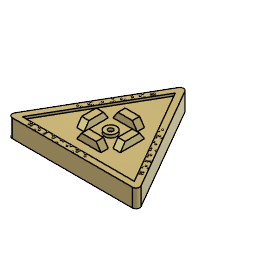
Piece Gold Minefinalweb (Autodesk Fusion 360 design; units mm, degrees)
Autodesk Fusion 360 part; units mm, degrees
note: some values were not read from the file. Set by a fixed rule: which sketch regions a step uses.
sketch "Sketch1" plane through (0, 0, 0) normal (0, 1, 0) x (1, 0, 0) in component "Goldmine"
  line L0 (0, 0) -> (69.85, 120.9837)
  line L1 (0, 0) -> (139.7, 0)
  line L2 (69.85, 120.9837) -> (139.7, 0)
  dimension "d1" = 139.7
  dimension "d2" = 139.7
  dimension "d4" = 139.7
  constraint coincident L0.start L1.start
  constraint horizontal L1
  measures "d1" distance of L0.start L0.end
  measures "d2" distance of L0.start L1.end
  measures "d4" distance of L0.end L1.end
extrude "Extrude1" add sketch "Sketch1" along normal blind 19.05 in component "Goldmine"
sketch "Sketch5" plane through (0, 19.05, 0) normal (0, 1, 0) x (-1, 0, 0) in component "Goldmine"
  line L0 (0, 0) -> (-139.7, 0)
  line L1 (-139.7, 0) -> (-69.85, -120.9837)
  line L2 (-69.85, -120.9837) -> (0, 0)
  line L3 (-10.9985, -6.35) -> (-69.85, -108.2837)
  line L4 (-69.85, -108.2837) -> (-128.7015, -6.35)
  line L5 (-128.7015, -6.35) -> (-10.9985, -6.35)
  dimension "d65" = 6.35
  dimension "d66" = 6.35
  dimension "d67" = 6.35
  constraint parallel L2 L3
  constraint parallel L1 L4
  constraint parallel L0 L5
  measures "d65" distance of L0 L3.start
  measures "d66" distance of L2 L3
  measures "d67" distance of L1 L4
extrude "Extrude6" cut sketch "Sketch5" against normal blind 2.54 contours L3 L4 L5 in component "Goldmine"
ref_plane "WorkPlane1" through (50.8, 0, 0) normal (1, 0, 0) x (0, 1, 0) in component "Goldmine"
sketch "Sketch10" plane through (0, 16.51, 0) normal (0, 1, 0) x (-1, 0, 0) in component "Goldmine"
  line L0 (-128.7015, -6.35) -> (-69.85, -108.2837)
  line L1 (-69.85, -108.2837) -> (-10.9985, -6.35)
  line L2 (-10.9985, -6.35) -> (-128.7015, -6.35)
  circle A0 centre (-69.85, -40.3279) radius 6.35
  circle A1 centre (-69.85, -40.3279) radius 2.54
  line L3 (-69.85, -40.3279) -> (-69.85, -108.2837) construction
  line L4 (-69.85, -40.3279) -> (-10.9985, -6.35) construction
  line L5 (-69.85, -40.3279) -> (-128.7015, -6.35) construction
  point P0 (-69.85, -108.2837)
  point P1 (-10.9985, -6.35)
  point P2 (-128.7015, -6.35)
  dimension "d125" = 12.7
  dimension "d126" = 5.08
  constraint concentric A0 A1
  constraint coincident A0.centre A1.centre
  constraint coincident P0 L0.end
  constraint coincident P1 L1.end
  constraint coincident P2 L0.start
  constraint equal L3 L4
  constraint equal L4 L5
  measures "d125" diameter of A0
  measures "d126" diameter of A1
extrude "Extrude14" add sketch "Sketch10" along normal blind 3.048 contours A0 in component "Goldmine"
sketch "Sketch11" plane through (0, 16.51, 0) normal (0, 1, 0) x (-1, 0, 0) in component "Goldmine"
  line L0 (-128.7015, -6.35) -> (-69.85, -108.2837)
  line L1 (-10.9985, -6.35) -> (-128.7015, -6.35)
  circle A0 centre (-69.85, -40.3279) radius 6.35
  circle A1 centre (-69.85, -40.3279) radius 2.54
  line L2 (-46.99, -53.0279) -> (-54.61, -53.0279)
  line L3 (-54.61, -53.0279) -> (-54.61, -27.6279)
  line L4 (-54.61, -27.6279) -> (-46.99, -27.6279)
  line L5 (-46.99, -27.6279) -> (-46.99, -53.0279)
  line L6 (-85.09, -53.0279) -> (-92.71, -53.0279)
  line L7 (-92.71, -53.0279) -> (-92.71, -27.6279)
  line L8 (-92.71, -27.6279) -> (-85.09, -27.6279)
  line L9 (-85.09, -27.6279) -> (-85.09, -53.0279)
  line L10 (-57.15, -63.1879) -> (-82.55, -63.1879)
  line L11 (-82.55, -63.1879) -> (-82.55, -55.5679)
  line L12 (-82.55, -25.0879) -> (-82.55, -17.4679)
  line L13 (-82.55, -17.4679) -> (-57.15, -17.4679)
  line L14 (-57.15, -63.1879) -> (-57.15, -55.5679)
  line L15 (-57.15, -55.5679) -> (-82.55, -55.5679)
  line L16 (-82.55, -25.0879) -> (-57.15, -25.0879)
  line L17 (-57.15, -25.0879) -> (-57.15, -17.4679)
  dimension "d129" = 25.4
  dimension "d130" = 7.62
  dimension "d131" = 15.24
  dimension "d132" = 12.7
  dimension "d133" = 7.62
  dimension "d134" = 25.4
  dimension "d135" = 30.48
  dimension "d152" = 2.54
  dimension "d153" = 7.62
  dimension "d154" = 25.4
  dimension "d155" = 7.62
  dimension "d156" = 15.24
  dimension "d157" = 2.54
  dimension "d158" = 7.62
  dimension "d159" = 25.4
  dimension "d160" = 15.24
  dimension "d161" = 2.54
  constraint horizontal L2
  constraint vertical L3
  constraint horizontal L4
  constraint vertical L5
  constraint horizontal L6
  constraint vertical L7
  constraint horizontal L8
  constraint vertical L9
  constraint horizontal L2.end L6.start
  constraint horizontal L10
  constraint vertical L11
  constraint vertical L12
  constraint horizontal L13
  constraint perpendicular L10 L14
  constraint perpendicular L3 L16
  constraint perpendicular L13 L17
  measures "d129" distance of L2.start L4.end
  measures "d130" distance of L3.end L4.end
  measures "d131" distance of A0.centre L3
  measures "d132" distance of A0.centre L2
  measures "d133" distance of L6.start L6.end
  measures "d134" distance of L6.start L8.end
  measures "d135" distance of L3 L9
  measures "d152" horizontal distance of L6.start L11.end
  measures "d153" distance of L10.end L11.end
  measures "d154" distance of L10.start L10.end
  measures "d155" distance of L10.start L14.end
  measures "d156" distance of A0.centre L15
  measures "d157" horizontal distance of L8.end L12.start
  measures "d158" distance of L12.start L12.end
  measures "d159" distance of L12.start L16.end
  measures "d160" vertical distance of A0.centre L16.end
  measures "d161" vertical distance of L8.end L12.start
extrude "Extrude15" add sketch "Sketch11" along normal blind 7.62 contours L2 L3 L4 L5 | L6 L7 L8 L9 | L10 L11 L14 L15 | L12 L13 L16 L17 in component "Goldmine"
sketch "Sketch12" plane through (92.71, 0, 0) normal (1, 0, 0) x (0, 0, -1) in component "Goldmine"
  line L0 (27.6279, 16.51) -> (53.0279, 16.51)
  line L1 (53.0279, 16.51) -> (53.0279, 24.13)
  line L2 (53.0279, 24.13) -> (27.6279, 24.13)
  line L3 (27.6279, 24.13) -> (27.6279, 16.51)
  line L4 (27.6279, 16.51) -> (32.7079, 24.13)
  line L5 (27.6279, 24.13) -> (27.6279, 16.51)
  line L6 (32.7079, 24.13) -> (27.6279, 24.13)
  line L7 (53.0279, 16.51) -> (47.9479, 24.13)
  line L8 (53.0279, 24.13) -> (47.9479, 24.13)
  line L9 (53.0279, 24.13) -> (53.0279, 16.51)
  dimension "d144" = 5.08
  dimension "d145" = 5.08
  constraint coincident L0.start L3.end
  constraint coincident L2 L4.end
  constraint coincident L2.end L3.start
  constraint coincident L0.end L1.start
  constraint coincident L2 L7.end
  constraint coincident L1.end L2.start
  measures "d144" distance of L7.end L1.end
  measures "d145" distance of L4.end L2.end
extrude "Extrude16" cut sketch "Sketch12" against normal blind 48.26 contours L2 L3 L4 L5 L6 | L1 L2 L7 L8 L9 in component "Goldmine"
sketch "Sketch13" plane through (0, 0, -17.4679) normal (0, 0, 1) x (1, 0, 0) in component "Goldmine"
  line L0 (57.15, 16.51) -> (82.55, 16.51)
  line L1 (82.55, 16.51) -> (82.55, 24.13)
  line L2 (82.55, 24.13) -> (57.15, 24.13)
  line L3 (57.15, 16.51) -> (62.23, 24.13)
  line L4 (62.23, 24.13) -> (57.15, 24.13)
  line L5 (57.15, 24.13) -> (57.15, 16.51)
  line L6 (82.55, 16.51) -> (77.47, 24.13)
  line L7 (77.47, 24.13) -> (82.55, 24.13)
  line L8 (82.55, 24.13) -> (82.55, 16.51)
  line L9 (57.15, 24.13) -> (57.15, 16.51)
  dimension "d148" = 5.08
  dimension "d149" = 5.08
  constraint coincident L0.start L3.start
  constraint coincident L2 L3.end
  constraint coincident L0.end L1.start
  constraint coincident L2 L6.end
  constraint coincident L1.end L2.start
  constraint coincident L2.end L4.end
  measures "d148" distance of L3.end L2.end
  measures "d149" distance of L6.end L1.end
extrude "Extrude17" cut sketch "Sketch13" against normal blind 55.88 contours L2 L3 L4 L5 L9 | L1 L2 L6 L7 L8 in component "Goldmine"
sketch "Sketch14" plane through (0, 19.05, 0) normal (0, 1, 0) x (-1, 0, 0) in component "Goldmine"
  line L0 (-10.9985, -6.35) -> (-69.85, -108.2837)
  line L1 (-69.85, -108.2837) -> (-128.7015, -6.35)
  line L2 (-128.7015, -6.35) -> (-10.9985, -6.35)
  line L3 (0, 0) -> (-139.7, 0)
  line L4 (-139.7, 0) -> (-69.85, -120.9837)
  line L5 (-69.85, -120.9837) -> (0, 0)
  circle A0 centre (-21.2442, -5.4189) radius 0.7493
  circle A1 centre (-21.2442, -3.1329) radius 0.7493
  circle A2 centre (-23.5302, -5.4189) radius 0.7493
  circle A3 centre (-23.5302, -3.1329) radius 0.7493
  circle A4 centre (-29.6516, -5.4189) radius 0.7493
  circle A5 centre (-31.9376, -3.1329) radius 0.7493
  circle A6 centre (-29.6516, -0.8469) radius 0.7493
  circle A7 centre (-38.059, -3.1329) radius 0.7493
  circle A8 centre (-38.059, -5.4189) radius 0.7493
  circle A9 centre (-38.059, -0.8469) radius 0.7493
  circle A10 centre (-44.1804, -5.4189) radius 0.7493
  circle A11 centre (-46.4664, -5.4189) radius 0.7493
  circle A12 centre (-46.4664, -3.1329) radius 0.7493
  circle A13 centre (-52.5878, -5.4189) radius 0.7493
  circle A14 centre (-54.8738, -5.4189) radius 0.7493
  circle A15 centre (-52.5878, -0.8469) radius 0.7493
  circle A16 centre (-60.9952, -3.1329) radius 0.7493
  circle A17 centre (-63.2812, -5.4189) radius 0.7493
  circle A18 centre (-69.4026, -5.4189) radius 0.7493
  circle A19 centre (-71.6886, -5.4189) radius 0.7493
  circle A20 centre (-71.6886, -3.1329) radius 0.7493
  circle A21 centre (-69.4026, -0.8469) radius 0.7493
  circle A22 centre (-77.81, -5.4189) radius 0.7493
  circle A23 centre (-80.096, -3.1329) radius 0.7493
  circle A24 centre (-124.1316, -16.0508) radius 0.7493
  circle A25 centre (-126.1113, -17.1938) radius 0.7493
  circle A26 centre (-122.9886, -18.0305) radius 0.7493
  circle A27 centre (-124.9683, -19.1735) radius 0.7493
  circle A28 centre (-119.9279, -23.3318) radius 0.7493
  circle A29 centre (-120.7646, -26.4545) radius 0.7493
  circle A30 centre (-123.8873, -25.6178) radius 0.7493
  circle A31 centre (-115.7242, -30.6128) radius 0.7493
  circle A32 centre (-117.7039, -31.7558) radius 0.7493
  circle A33 centre (-119.6836, -32.8988) radius 0.7493
  circle A34 centre (-112.6635, -35.9141) radius 0.7493
  circle A35 centre (-111.5205, -37.8938) radius 0.7493
  circle A36 centre (-113.5002, -39.0368) radius 0.7493
  circle A37 centre (-108.4598, -43.1951) radius 0.7493
  circle A38 centre (-112.4192, -45.4811) radius 0.7493
  circle A39 centre (-107.3168, -45.1749) radius 0.7493
  circle A40 centre (-106.2358, -51.6192) radius 0.7493
  circle A41 centre (-103.1131, -52.4559) radius 0.7493
  circle A42 centre (-100.0524, -57.7572) radius 0.7493
  circle A43 centre (-98.9094, -59.7369) radius 0.7493
  circle A44 centre (-100.8891, -60.8799) radius 0.7493
  circle A45 centre (-95.8487, -65.0382) radius 0.7493
  circle A46 centre (-96.6854, -68.1609) radius 0.7493
  circle A47 centre (-104.0118, -60.0432) radius 0.7493
  circle A48 centre (-61.3723, -95.4278) radius 0.7493
  circle A49 centre (-59.3926, -96.5708) radius 0.7493
  circle A50 centre (-60.2293, -93.448) radius 0.7493
  circle A51 centre (-58.2496, -94.591) radius 0.7493
  circle A52 centre (-57.1686, -88.1468) radius 0.7493
  circle A53 centre (-54.0459, -87.31) radius 0.7493
  circle A54 centre (-53.2091, -90.4328) radius 0.7493
  circle A55 centre (-52.9649, -80.8657) radius 0.7493
  circle A56 centre (-50.9852, -82.0087) radius 0.7493
  circle A57 centre (-49.0054, -83.1517) radius 0.7493
  circle A58 centre (-49.9042, -75.5644) radius 0.7493
  circle A59 centre (-48.7612, -73.5847) radius 0.7493
  circle A60 centre (-46.7815, -74.7277) radius 0.7493
  circle A61 centre (-45.7005, -68.2834) radius 0.7493
  circle A62 centre (-41.741, -70.5694) radius 0.7493
  circle A63 centre (-44.5575, -66.3037) radius 0.7493
  circle A64 centre (-39.5171, -62.1454) radius 0.7493
  circle A65 centre (-40.3538, -59.0227) radius 0.7493
  circle A66 centre (-37.2931, -53.7214) radius 0.7493
  circle A67 centre (-36.1501, -51.7416) radius 0.7493
  circle A68 centre (-34.1704, -52.8846) radius 0.7493
  circle A69 centre (-33.0894, -46.4404) radius 0.7493
  circle A70 centre (-29.9667, -45.6036) radius 0.7493
  circle A71 centre (-33.3336, -56.0074) radius 0.7493
  dimension "d162" = 1.4986
  dimension "d163" = 1.4986
  dimension "d165" = 1.4986
  dimension "d166" = 1.4986
  dimension "d167" = 1.4986
  dimension "d168" = 1.4986
  dimension "d169" = 1.4986
  dimension "d170" = 1.4986
  dimension "d171" = 1.4986
  dimension "d172" = 1.4986
  dimension "d173" = 1.4986
  dimension "d174" = 1.4986
  dimension "d175" = 1.4986
  dimension "d176" = 1.4986
  dimension "d177" = 1.4986
  dimension "d178" = 1.4986
  dimension "d180" = 1.4986
  dimension "d181" = 1.4986
  dimension "d182" = 1.4986
  dimension "d183" = 1.4986
  dimension "d184" = 1.4986
  dimension "d185" = 1.4986
  dimension "d186" = 1.4986
  dimension "d187" = 1.4986
  dimension "d188" = 1.4986
  dimension "d189" = 1.4986
  dimension "d190" = 1.4986
  dimension "d191" = 1.4986
  dimension "d192" = 1.4986
  dimension "d193" = 1.4986
  dimension "d194" = 1.4986
  dimension "d195" = 1.4986
  dimension "d196" = 1.4986
  dimension "d197" = 1.4986
  dimension "d198" = 1.4986
  dimension "d199" = 1.4986
  dimension "d200" = 1.4986
  dimension "d201" = 1.4986
  dimension "d202" = 1.4986
  dimension "d203" = 1.4986
  dimension "d204" = 1.4986
  dimension "d205" = 1.4986
  dimension "d206" = 1.4986
  dimension "d207" = 1.4986
  dimension "d208" = 1.4986
  dimension "d209" = 1.4986
  dimension "d210" = 1.4986
  dimension "d211" = 1.4986
  dimension "d212" = 1.4986
  dimension "d213" = 1.4986
  dimension "d214" = 1.4986
  dimension "d215" = 1.4986
  dimension "d216" = 1.4986
  dimension "d217" = 1.4986
  dimension "d218" = 1.4986
  dimension "d219" = 1.4986
  dimension "d220" = 1.4986
  dimension "d221" = 1.4986
  dimension "d222" = 1.4986
  dimension "d223" = 1.4986
  dimension "d224" = 1.4986
  dimension "d225" = 1.4986
  dimension "d226" = 1.4986
  dimension "d227" = 1.4986
  dimension "d228" = 1.4986
  dimension "d229" = 1.4986
  dimension "d230" = 1.4986
  dimension "d231" = 1.4986
  dimension "d232" = 1.4986
  dimension "d233" = 1.4986
  dimension "d234" = 1.4986
  dimension "d235" = 1.4986
  measures "d162" diameter of A0
  measures "d163" diameter of A1
  measures "d165" diameter of A2
  measures "d166" diameter of A3
  measures "d167" diameter of A4
  measures "d168" diameter of A5
  measures "d169" diameter of A6
  measures "d170" diameter of A7
  measures "d171" diameter of A8
  measures "d172" diameter of A9
  measures "d173" diameter of A10
  measures "d174" diameter of A11
  measures "d175" diameter of A12
  measures "d176" diameter of A13
  measures "d177" diameter of A14
  measures "d178" diameter of A15
  measures "d180" diameter of A16
  measures "d181" diameter of A17
  measures "d182" diameter of A18
  measures "d183" diameter of A19
  measures "d184" diameter of A20
  measures "d185" diameter of A21
  measures "d186" diameter of A22
  measures "d187" diameter of A23
  measures "d188" diameter of A24
  measures "d189" diameter of A25
  measures "d190" diameter of A26
  measures "d191" diameter of A27
  measures "d192" diameter of A28
  measures "d193" diameter of A29
  measures "d194" diameter of A30
  measures "d195" diameter of A32
  measures "d196" diameter of A31
  measures "d197" diameter of A33
  measures "d198" diameter of A34
  measures "d199" diameter of A35
  measures "d200" diameter of A36
  measures "d201" diameter of A37
  measures "d202" diameter of A39
  measures "d203" diameter of A38
  measures "d204" diameter of A40
  measures "d205" diameter of A41
  measures "d206" diameter of A42
  measures "d207" diameter of A43
  measures "d208" diameter of A44
  measures "d209" diameter of A47
  measures "d210" diameter of A45
  measures "d211" diameter of A46
  measures "d212" diameter of A48
  measures "d213" diameter of A49
  measures "d214" diameter of A50
  measures "d215" diameter of A51
  measures "d216" diameter of A52
  measures "d217" diameter of A53
  measures "d218" diameter of A54
  measures "d219" diameter of A56
  measures "d220" diameter of A55
  measures "d221" diameter of A57
  measures "d222" diameter of A58
  measures "d223" diameter of A59
  measures "d224" diameter of A60
  measures "d225" diameter of A61
  measures "d226" diameter of A63
  measures "d227" diameter of A62
  measures "d228" diameter of A64
  measures "d229" diameter of A65
  measures "d230" diameter of A66
  measures "d231" diameter of A67
  measures "d232" diameter of A68
  measures "d233" diameter of A71
  measures "d234" diameter of A69
  measures "d235" diameter of A70
extrude "Extrude18" add sketch "Sketch14" along normal blind 0.762 contours A0 | A1 | A2 | A3 | A4 | A5 | A6 | A7 | A8 | A9 | A10 | A11 | A12 | A13 | A14 | A15 | A16 | A17 | A18 | A19 | A20 | A21 | A22 | A23 | A24 | A25 | A26 | A27 | A28 | A29 | A30 | A31 | A32 | A33 | A34 | A35 | A36 | A37 | A38 | A39 | A40 | A41 | A42 | A43 | A44 | A45 | A46 | A47 | A48 | A49 | A50 | A51 | A52 | A53 | A54 | A55 | A56 | A57 | A58 | A59 | A60 | A61 | A62 | A63 | A64 | A65 | A66 | A67 | A68 | A69 | A70 | A71 in component "Goldmine"
fillet "Fillet1" radius 0.7493 72 edges at (21.9428, 19.812, -5.6899) (24.2288, 19.812, -5.6899) (24.2288, 19.812, -3.4039) (21.9428, 19.812, -3.4039) (32.6362, 19.812, -3.4039) (30.3502, 19.812, -5.6899) (30.3502, 19.812, -1.1179) (38.7576, 19.812, -5.6899) (38.7576, 19.812, -3.4039) (38.7576, 19.812, -1.1179) (47.165, 19.812, -5.6899) (47.165, 19.812, -3.4039) (44.879, 19.812, -5.6899) (53.2864, 19.812, -5.6899) (53.2864, 19.812, -1.1179) (55.5724, 19.812, -5.6899) (61.6938, 19.812, -3.4039) (63.9798, 19.812, -5.6899) (78.5086, 19.812, -5.6899) (80.7946, 19.812, -3.4039) (72.3872, 19.812, -5.6899) (72.3872, 19.812, -3.4039) (70.1012, 19.812, -5.6899) (70.1012, 19.812, -1.1179) (123.5476, 19.812, -16.5203) (124.3844, 19.812, -19.643) (125.5274, 19.812, -17.6633) (122.4046, 19.812, -18.5) (120.1807, 19.812, -26.9241) (123.3034, 19.812, -26.0873) (119.3439, 19.812, -23.8013) (115.1402, 19.812, -31.0823) (117.12, 19.812, -32.2253) (119.0997, 19.812, -33.3683) (112.0795, 19.812, -36.3836) (112.9163, 19.812, -39.5064) (110.9365, 19.812, -38.3634) (96.1015, 19.812, -68.6305) (95.2647, 19.812, -65.5077) (100.3052, 19.812, -61.3494) (103.4279, 19.812, -60.5127) (98.3254, 19.812, -60.2064) (99.4684, 19.812, -58.2267) (102.5291, 19.812, -52.9254) (105.6519, 19.812, -52.0887) (111.8353, 19.812, -45.9507) (106.7328, 19.812, -45.6444) (107.8758, 19.812, -43.6647) (59.2779, 19.812, -95.8303) (61.2577, 19.812, -94.6873) (60.1147, 19.812, -92.7076) (58.1349, 19.812, -93.8506) (57.054, 19.812, -87.4063) (53.0945, 19.812, -89.6923) (53.9312, 19.812, -86.5695) (48.8908, 19.812, -82.4113) (50.8705, 19.812, -81.2683) (52.8503, 19.812, -80.1253) (46.6668, 19.812, -73.9872) (49.7896, 19.812, -74.824) (48.6466, 19.812, -72.8442) (45.5859, 19.812, -67.5429) (44.4429, 19.812, -65.5632) (41.6264, 19.812, -69.8289) (39.4024, 19.812, -61.4049) (40.2392, 19.812, -58.2822) (37.1785, 19.812, -52.9809) (36.0355, 19.812, -51.0012) (34.0557, 19.812, -52.1442) (33.219, 19.812, -55.2669) (32.9748, 19.812, -45.6999) (29.852, 19.812, -44.8631) in component "Goldmine"
fillet "Fillet2" radius 3.81 3 edges at (139.7, 9.525, 0) (0, 9.525, 0) (69.85, 9.525, -120.9837) in component "Goldmine"
component "Goldmine" placed x (1, 0, 0) y (0, 1, 0) z (0, 0, 1) at (0, 0, 0)
